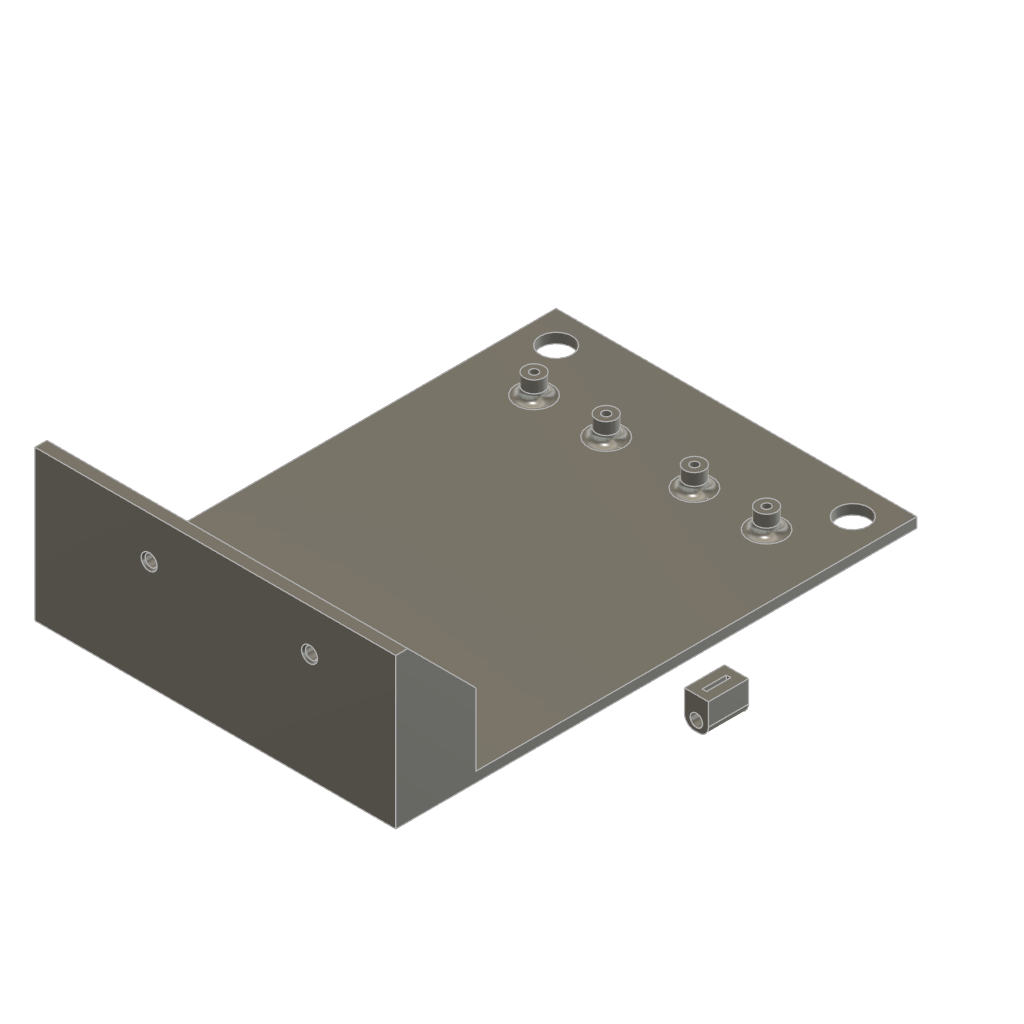
Throttle +MIX (Autodesk Fusion 360 design; units mm, degrees)
Autodesk Fusion 360 part; units mm, degrees
sketch "Sketch1" plane through (0, 0, 0) normal (0, 1, 0) x (1, 0, 0)
  line L0 (-9.5, -45) -> (-30.5, -45) construction
  line L1 (-30.5, -45) -> (-30.5, 45) construction
  line L2 (-30.5, 45) -> (-9.5, 45) construction
  line L3 (-9.5, 45) -> (-9.5, -45) construction
  line L4 (-9.5, -45) -> (-30.5, 45) construction
  line L5 (-30.5, -45) -> (-9.5, 45) construction
  circle A0 centre (-29, 43.5) radius 1.5
  circle A1 centre (-11, 43.5) radius 1.5
  circle A2 centre (-29, -43.5) radius 1.5
  circle A3 centre (-11, -43.5) radius 1.5
  circle A4 centre (-29, 43.5) radius 1
  circle A5 centre (-11, 43.5) radius 1
  circle A6 centre (-29, -43.5) radius 1
  circle A7 centre (-11, -43.5) radius 1
  circle A8 centre (-29, 43.5) radius 2.5
  circle A9 centre (-11, 43.5) radius 2.5
  circle A10 centre (-29, -43.5) radius 2.5
  circle A11 centre (-11, -43.5) radius 2.5
  line L6 (0, 70) -> (0, -70) construction
  circle A12 centre (29, 43.5) radius 1.5
  circle A13 centre (11, -43.5) radius 1
  circle A14 centre (29, 43.5) radius 1
  line L7 (30.5, -45) -> (30.5, 45) construction
  circle A15 centre (29, 43.5) radius 2.5
  circle A16 centre (11, 43.5) radius 2.5
  circle A17 centre (11, -43.5) radius 2.5
  line L8 (9.5, 45) -> (9.5, -45) construction
  circle A18 centre (29, -43.5) radius 2.5
  line L9 (30.5, 45) -> (9.5, 45) construction
  circle A19 centre (11, -43.5) radius 1.5
  circle A20 centre (29, -43.5) radius 1
  line L10 (9.5, -45) -> (30.5, 45) construction
  circle A21 centre (11, 43.5) radius 1.5
  circle A22 centre (29, -43.5) radius 1.5
  line L11 (9.5, -45) -> (30.5, -45) construction
  line L12 (30.5, -45) -> (9.5, 45) construction
  circle A23 centre (11, 43.5) radius 1
  line L13 (45, -65) -> (-45, -65)
  line L14 (-45, -65) -> (-45, 65)
  line L15 (-45, 65) -> (45, 65)
  line L16 (45, 65) -> (45, -65)
  line L17 (45, -65) -> (-45, 65) construction
  line L18 (-45, -65) -> (45, 65) construction
  circle A24 centre (-37, 57) radius 8
  circle A25 centre (-37, 57) radius 4
  line L19 (-45, 0) -> (45, 0) construction
  circle A26 centre (37, 57) radius 8
  circle A27 centre (37, 57) radius 4
  point P0 (-20, 0)
  point P1 (20, 0)
  dimension "d1" = 21
  dimension "d2" = 90
  dimension "d3" = 20
  dimension "d4" = 1.5
  dimension "d5" = 1.5
  dimension "d6" = 1.5
  dimension "d7" = 1.5
  dimension "d8" = 2
  dimension "d9" = 2
  dimension "d10" = 2
  dimension "d11" = 2
  dimension "d12" = 1
  dimension "d13" = 1
  dimension "d14" = 1
  dimension "d15" = 1
  dimension "d16" = 90
  dimension "d17" = 130
  dimension "d18" = 8
  dimension "d19" = -4
  dimension "d22" = 1.5
  constraint horizontal L0
  constraint perpendicular L0 L1
  constraint parallel L0 L2
  constraint parallel L1 L3
  constraint coincident L4 P0
  constraint coincident L5 P0
  constraint tangent L2 A0
  constraint tangent L1 A0
  constraint tangent L2 A1
  constraint tangent L3 A1
  constraint tangent L1 A2
  constraint tangent L0 A2
  constraint tangent L3 A3
  constraint tangent L0 A3
  constraint concentric A0 A4
  constraint concentric A1 A5
  constraint concentric A2 A6
  constraint concentric A3 A7
  constraint vertical L6
  constraint symmetric L0.start L6 L8.end
  constraint symmetric L0.end L6 L7.start
  constraint symmetric L1.end L6 L7.end
  constraint symmetric L2.end L6 L8.start
  constraint symmetric P0 L6 P1
  constraint symmetric A0 L6 A12
  constraint symmetric A1 L6 A21
  constraint symmetric A2 L6 A22
  constraint symmetric A3 L6 A19
  constraint symmetric A4 L6 A14
  constraint symmetric A5 L6 A23
  constraint symmetric A6 L6 A20
  constraint symmetric A7 L6 A13
  constraint symmetric A8 L6 A15
  constraint symmetric A9 L6 A16
  constraint symmetric A10 L6 A18
  constraint symmetric A11 L6 A17
  constraint horizontal L13
  constraint perpendicular L13 L14
  constraint parallel L13 L15
  constraint parallel L14 L16
  constraint coincident L17 origin
  constraint coincident L18 origin
  constraint tangent L15 A24
  constraint tangent L14 A24
  constraint midpoint L14 L19.start
  constraint midpoint L16 L19.end
  constraint symmetric L6 A24 A26
  constraint symmetric L6 A25 A27
  measures "d1" distance of L1.end L2.end
  measures "d2" distance of L0.end L1.end
  measures "d3" distance of origin P0
  measures "d4" radius of A0
  measures "d5" radius of A1
  measures "d6" radius of A2
  measures "d7" radius of A3
  measures "d8" diameter of A4
  measures "d9" diameter of A5
  measures "d10" diameter of A6
  measures "d11" diameter of A7
  measures "d16" distance of L14.end L15.end
  measures "d17" distance of L13.end L14.end
  measures "d18" radius of A24
  measures "d22" distance of A6 A10
extrude "Extrude1" add sketch "Sketch1" against normal blind 2.5 contours A0 | A1 | A2 | A3 | A4 | A5 | A6 | A7 | A8 | A9 | A10 | A11 | A12 | A13 | A14 | A15 | A16 | A17 | A18 | A19 | A20 | A21 | A22 | A23 | L13 L14 L15 L16 A24 A26 | L15 L16 A26 | A26 | L14 L15 A24 | A24 makes body 1
extrude "Extrude2" add sketch "Sketch1" along normal blind 5 contours A0 | A1 | A2 | A3 | A8 | A9 | A10 | A11 | A12 | A15 | A16 | A17 | A18 | A19 | A21 | A22 bodies 1
sketch "Sketch2" plane through (0, 0, 0) normal (0, 1, 0) x (-1, 0, 0)
  circle A0 centre (-29, -43.5) radius 2.5
  circle A1 centre (11, 43.5) radius 2.5
  circle A2 centre (-11, -43.5) radius 2.5
  circle A3 centre (29, 43.5) radius 2.5
  circle A4 centre (-37, -57) radius 4
  circle A5 centre (37, -57) radius 4
  line L0 (-45, -65) -> (45, -65)
  line L1 (45, -65) -> (45, 65)
  line L2 (45, 65) -> (-45, 65)
  line L3 (-45, 65) -> (-45, -65)
  circle A6 centre (11, -43.5) radius 2.5
  circle A7 centre (-11, 43.5) radius 2.5
  circle A8 centre (29, -43.5) radius 2.5
  circle A9 centre (-29, 43.5) radius 2.5
  line L4 (45, 65) -> (-45, 65)
  line L5 (-45, 65) -> (-45, 62)
  line L6 (-45, 62) -> (45, 62)
  line L7 (45, 62) -> (45, 65)
  line L8 (45, 65) -> (42, 65)
  line L9 (42, 65) -> (42, 45)
  line L10 (42, 45) -> (45, 45)
  line L11 (45, 45) -> (45, 65)
  line L12 (-45, 65) -> (-42, 65)
  line L13 (-42, 65) -> (-42, 45)
  line L14 (-42, 45) -> (-45, 45)
  line L15 (-45, 45) -> (-45, 65)
  dimension "d25" = 90
  dimension "d26" = 3
  dimension "d27" = 3
  dimension "d28" = 20
  dimension "d31" = 3
  constraint horizontal L4
  constraint vertical L5
  constraint horizontal L6
  constraint vertical L7
  constraint coincident L1.end L2.start
  constraint horizontal L8
  constraint vertical L9
  constraint horizontal L10
  constraint vertical L11
  constraint horizontal L12
  constraint vertical L13
  constraint horizontal L14
  constraint vertical L15
  constraint coincident L2.end L3.start
  measures "d25" distance of L1.end L2.end
  measures "d26" distance of L1.end L6.end
  measures "d27" distance of L2.end L12.end
  measures "d28" distance of L2.end L14.end
  measures "d31" distance of L9.end L10.end
extrude "Extrude3" add sketch "Sketch2" along normal blind 35 contours L3 L6 L13 L14 L15 | L1 L6 L9 L10 L11 | L2 L3 L4 L5 L6 L12 L13 L15 | L1 L2 L4 L6 L7 L8 L9 L11 | L2 L4 L6 L9 L13 bodies 1
chamfer "Chamfer1" distance 17 angle 45 2 edges at (-43.5, 35, 45) (43.5, 35, 45) on bodies 1
hole "Hole1" at (-16.5, 24.5, 65) direction (0, 0, -1) diameter 3 depth 5 tip angle 118 bodies 1
hole "Hole2" at (23.5, 24.5, 65) direction (0, 0, -1) diameter 3 depth 5 tip angle 118 bodies 1
fillet "Fillet1" radius 5 3 edges at (0, 0, 62) (42, 0, 53.5) (-42, 0, 53.5) on bodies 1
chamfer "Chamfer2" distance 0.5 angle 45 4 edges at (-17.8985, 25.0424, 65) (-17.8985, 23.9576, 62) (22.1015, 25.0424, 65) (22.1015, 23.9576, 62) on bodies 1
sketch "Sketch3" plane through (0, 0, 0) normal (0, 1, 0) x (1, 0, 0)
  line L0 (3, 5) -> (-3, 5)
  line L1 (-3, 5) -> (-3, -5)
  line L2 (-3, -5) -> (3, -5)
  line L3 (3, -5) -> (3, 5)
  line L4 (3, 5) -> (-3, -5) construction
  line L5 (-3, 5) -> (3, -5) construction
  line L6 (0.55, -3) -> (-0.55, -3)
  line L7 (-0.55, -3) -> (-0.55, 3)
  line L8 (-0.55, 3) -> (0.55, 3)
  line L9 (0.55, 3) -> (0.55, -3)
  line L10 (0.55, -3) -> (-0.55, 3) construction
  line L11 (-0.55, -3) -> (0.55, 3) construction
  dimension "d46" = 6
  dimension "d47" = 10
  dimension "d48" = 1.1
  dimension "d49" = 6
  constraint horizontal L0
  constraint perpendicular L0 L1
  constraint parallel L0 L2
  constraint parallel L1 L3
  constraint coincident L4 origin
  constraint coincident L5 origin
  constraint horizontal L6
  constraint perpendicular L6 L7
  constraint parallel L6 L8
  constraint parallel L7 L9
  constraint coincident L10 origin
  constraint coincident L11 origin
  measures "d46" distance of L1.end L2.end
  measures "d47" distance of L0.end L1.end
  measures "d48" distance of L7.end L8.end
  measures "d49" distance of L6.end L7.end
extrude "Extrude4" add sketch "Sketch3" against normal blind 4 separate body contours L0 L1 L2 L3 | L6 L7 L8 L9 makes body 2
extrude "Extrude5" add sketch "Sketch3" along normal blind 4 bodies 2
fillet "Fillet2" radius 2.5 2 edges at (3, -4, 0) (-3, -4, 0) on bodies 2
hole "Hole3" at (0, -1.5, -5) direction (0, 0, 1) diameter 3.1 depth 10 tip angle 118 bodies 2
move_body "Move1" bodies 2 to x (1, 0, 0) y (0, 1, 0) z (0, 0, 1) at (60, 0, 0)
fillet "Fillet3" radius 2 8 edges at (26.6692, 0, 42.596) (8.6692, 0, 42.596) (-13.3308, 0, 42.596) (-31.3308, 0, 42.596) (-31.3308, 0, -44.404) (-13.3308, 0, -44.404) (8.6692, 0, -44.404) (26.6692, 0, -44.404) on bodies 1
